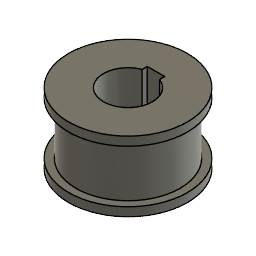
_Nema 34 Pulley HTD 3M x 15.26af3756-7a5c-4958-96f5-3b08fcf63012 (Autodesk Fusion 360 design; units mm, degrees)
Autodesk Fusion 360 part; units mm, degrees
sketch "Sketch1" plane through (0, 0, 0) normal (0, 1, 0) x (1, 0, 0)
  circle A0 centre (0, 0) radius 17
  circle A1 centre (0, 0) radius 14.895
  line L0 (0, 0) -> (0, 8) construction
  line L1 (0, 8) -> (2.5, 8)
  line L2 (2.5, 8) -> (2.5, 6.5383)
  line L3 (0, 8) -> (-2.5, 8)
  line L4 (-2.5, 8) -> (-2.5, 6.5383)
  arc A2 (-2.5, 6.5383) -> (2.5, 6.5383) centre (0, 0) ccw
  dimension "d1" = 34
  dimension "d2" = 29.79
  dimension "d3" = 14
  dimension "d4" = 2.5
  dimension "d5" = 2.5
  dimension "d6" = 8
  constraint coincident A0.centre A1.centre
  constraint concentric A0 A1
  constraint concentric A1 A2
  constraint vertical L0
  constraint perpendicular L0 L1
  constraint perpendicular L1 L2
  constraint perpendicular L0 L3
  constraint perpendicular L3 L4
  measures "d1" diameter of A0
  measures "d2" diameter of A1
  measures "d3" diameter of A2
  measures "d4" distance of L0.end L1.end
  measures "d5" distance of L0.end L3.end
  measures "d6" distance of A0.centre L0.end
extrude "Extrude1" add sketch "Sketch1" against normal blind 2.5 contours A0 | A1
extrude "Extrude2" add sketch "Sketch1" along normal blind 15 contours A1
extrude "Extrude3" add sketch "Sketch1" along normal blind 2.5 from surface at 15 contours A0 | A1
